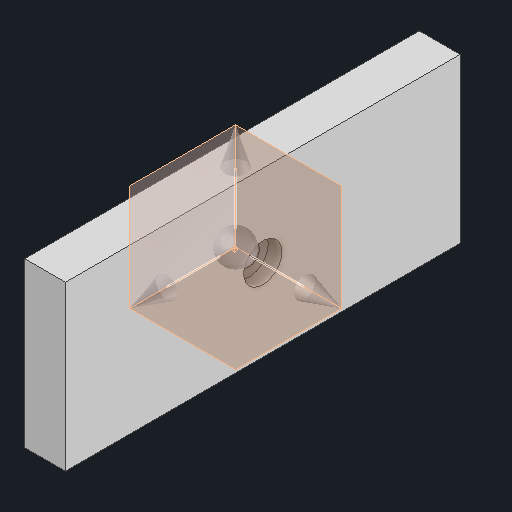
# Autodesk Inventor part: Vertical Spinner Weapon V3
Saved by Autodesk Inventor 2026.2 (Build 302298000, 298)
## iProperties
Created: 2023-08-18
Part Number: Vertical Spinner Weapon V3
Material: Generic
Document SubType Name: Modeling
Designer: vandj
Density: 1 g/cm^3
Appearance: Default
Mass: 70.3924 g
Surface Area: 175.698 cm^2
Volume: 70.3924 cm^3
Author: vandj
Autodesk Inventor part; units mm, degrees
ref_plane "YZ Plane" through (0, 0, 0) normal (1, 0, 0) x (0, 1, 0)
ref_plane "XZ Plane" through (0, 0, 0) normal (0, 1, 0) x (-1, 0, 0)
ref_plane "XY Plane" through (0, 0, 0) normal (0, 0, 1) x (1, 0, 0)
sketch "Sketch 1" plane through (0, 0, 0) normal (1, 0, 0) x (0, 1, 0)
  circle A0 centre (0, 0) radius 2.5
  circle A1 centre (0, 0) radius 25
  point P0 (1.2916, -31.2195)
  point P1 (0, 30.3272)
  point P2 (-0.1255, 30.3272)
  point P3 (0, -30.3272)
  point P4 (0.1231, -30.3272)
  point P5 (-1.2948, 31.2193)
  point P6 (0.0032, -40.9065)
  point P7 (0, -40.9065)
  point P8 (-1.4137, 30.3272)
  dimension "d22" = 5
  dimension "d51" = 50
  constraints: 2 centre point, 2 coincident
  measures "d22" diameter of A0
  measures "d51" diameter of A1
extrude "Interface" add sketch "Sketch 1" along normal blind 15
sketch "Sketch9" plane through (0, 0, 0) normal (-1, 0, 0) x (0, 0, 1)
  circle A0 centre (0, 0) radius 2.5 projected
  circle A1 centre (0, 0) radius 3.75
  dimension "d32" = 7.5
  constraints: 1 centre point, 1 coincident
  measures "d32" diameter of A1
extrude "Shaft Hole" cut sketch "Sketch9" against normal blind 28.1375
sketch "Sketch10" plane through (15, 0, 0) normal (1, 0, 0) x (0, 0, -1)
  circle A0 centre (0, 0) radius 3.75 projected
  circle A1 centre (0, 0) radius 7
  dimension "d35" = 14
  constraints: 1 centre point, 1 coincident
  measures "d35" diameter of A1
extrude "Bearing Hole" cut sketch "Sketch10" against normal blind 5
sketch "EDIT WEAPON SKETCH" plane through (0, 0, 0) normal (1, 0, 0) x (0, 1, 0)
  circle A0 centre (0, 0) radius 25 projected
  circle A1 centre (0, 0) radius 25 projected
  line L0 (83.5575, 140.0168) -> (83.5575, 44.1301) construction
  line L1 (83.5575, 44.1301) -> (66.7631, 44.1301) construction
  line L2 (66.7631, 44.1301) -> (66.7631, 140.0168) construction
  line L3 (66.7631, 140.0168) -> (83.5575, 140.0168) construction
  line L4 (-30.0586, 72.5) -> (30.0586, 72.5)
  line L5 (30.0586, 72.5) -> (30.0586, -72.5)
  line L6 (30.0586, -72.5) -> (-30.0586, -72.5)
  line L7 (-30.0586, -72.5) -> (-30.0586, 72.5)
  circle A2 centre (0, 0) radius 3.75 projected
  line L8 (-30.0586, 72.5) -> (30.0586, -72.5) construction
  line L9 (30.0586, 72.5) -> (-30.0586, -72.5) construction
  constraints: 12 end point, 2 midpoint, 2 parallel, 1 horizontal, 1 perpendicular, 2 other
extrude "EDIT WEAPON SHAPE" add sketch "EDIT WEAPON SKETCH" along normal up to surface (15 mm away) contours L4 L5 L6 L7
body "Solid1"
